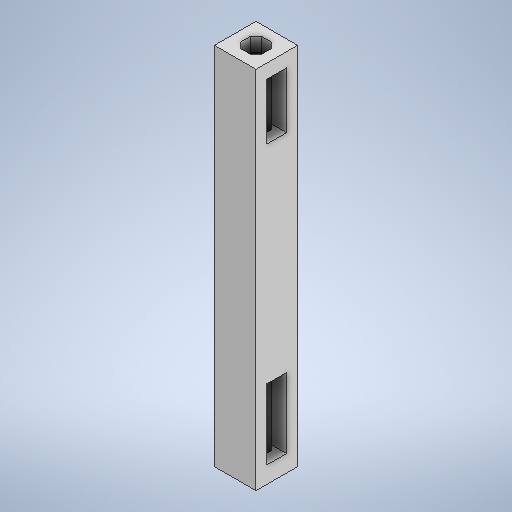
# Autodesk Inventor part: Square Supports
Saved by Autodesk Inventor 2026.2 (Build 302298010, 298A)
## iProperties
Created: 2026-05-07
Part Number: Square Supports
Material: Generic
Document SubType Name: Modeling
Designer: piete
Density: 1 g/cm^3
Appearance: Default
Author: piete
Autodesk Inventor part; units mm, degrees
ref_plane "YZ Plane" through (0, 0, 0) normal (1, 0, 0) x (0, 1, 0)
ref_plane "XZ Plane" through (0, 0, 0) normal (0, 1, 0) x (-1, 0, 0)
ref_plane "XY Plane" through (0, 0, 0) normal (0, 0, 1) x (1, 0, 0)
sketch "Sketch1" plane through (0, 0, 0) normal (0, 1, 0) x (-1, 0, 0)
  line L0 (7.4, 7.4) -> (-7.4, 7.4)
  line L1 (-7.4, 7.4) -> (-7.4, -7.4)
  line L2 (-7.4, -7.4) -> (7.4, -7.4)
  line L3 (7.4, -7.4) -> (7.4, 7.4)
  point P0 (0, 0)
  dimension "d0" = 14.8
  dimension "d1" = 14.8
  dimension "d2" = 7.4
  dimension "d3" = 7.4
  constraints: 8 end point, 2 parallel, 1 horizontal, 1 perpendicular
  measures "d0" distance of L2.end L1.end
  measures "d1" distance of L2.end L0.start
  measures "d2" distance from line of point (0, 0) L3
  measures "d3" distance from line of point (0, 0) L2
extrude "Extrusion1" add sketch "Sketch1" along normal blind 130
sketch "Sketch2" plane through (7.4, 0, 7.4) normal (1, 0, 0) x (0, 0, -1)
  line L0 (3.9, 31) -> (10.9, 31)
  line L1 (10.9, 31) -> (10.9, 6)
  line L2 (10.9, 6) -> (3.9, 6)
  line L3 (3.9, 6) -> (3.9, 31)
  line L4 (0, 0) -> (14.8, 0) projected
  line L5 (3.9, 125) -> (10.9, 125)
  line L6 (10.9, 125) -> (10.9, 105)
  line L7 (10.9, 105) -> (3.9, 105)
  line L8 (3.9, 105) -> (3.9, 125)
  line L9 (0, 130) -> (14.8, 130) projected
  point P0 (7.4, 0)
  point P1 (7.4, 0)
  point P2 (7.4, 6)
  point P3 (7.4, 0)
  point P4 (7.4, 130)
  point P5 (7.4, 125)
  dimension "d6" = 7
  dimension "d7" = 25
  dimension "d8" = 6
  dimension "d9" = 0
  dimension "d10" = 7
  dimension "d11" = 20
  dimension "d12" = 0
  dimension "d14" = 119
  constraints: 16 end point, 5 midpoint, 4 parallel, 2 horizontal, 2 perpendicular
  measures "d6" distance of L1.end L2.end
  measures "d7" distance of L0.end L1.end
  measures "d8" distance of point (7.4, 0) point (7.4, 6)
  measures "d9" horizontal distance of point (7.4, 0) point (7.4, 6)
  measures "d10" distance of L6.end L7.end
  measures "d11" distance of L5.end L6.end
  measures "d12" horizontal distance of point (7.4, 130) point (7.4, 125)
  measures "d14" distance between parallel lines of L2 L5
extrude "Extrusion2" cut sketch "Sketch2" against normal through all
sketch "Sketch3" plane through (0, 130, 0) normal (0, 1, 0) x (1, 0, 0)
  line L0 (-3.75, -3.75) -> (3.75, -3.75)
  line L1 (3.75, -3.75) -> (3.75, 3.75)
  line L2 (3.75, 3.75) -> (-3.75, 3.75)
  line L3 (-3.75, 3.75) -> (-3.75, -3.75)
  point P0 (0, 0)
  dimension "d17" = 7.5
  dimension "d18" = 7.5
  dimension "d19" = 3.75
  dimension "d20" = 3.75
  constraints: 8 end point, 2 parallel, 1 horizontal, 1 perpendicular
  measures "d17" distance of L2.end L1.end
  measures "d18" distance of L1.end L0.end
  measures "d19" distance from line of point (0, 0) L3
  measures "d20" distance from line of point (0, 0) L2
extrude "Extrusion3" cut sketch "Sketch3" against normal through all
chamfer "Chamfer1" distance 2 angle 45 4 edges at (-3.75, 65, -3.75) (3.75, 65, -3.75) (-3.75, 65, 3.75) (3.75, 65, 3.75)
equation "\"d2\" = 0.5 * d0"
equation "\"d3\" = 0.5 * d1"
equation "\"d19\" = 0.5 * d17"
equation "\"d20\" = 0.5 * d18"
body "Solid1"
